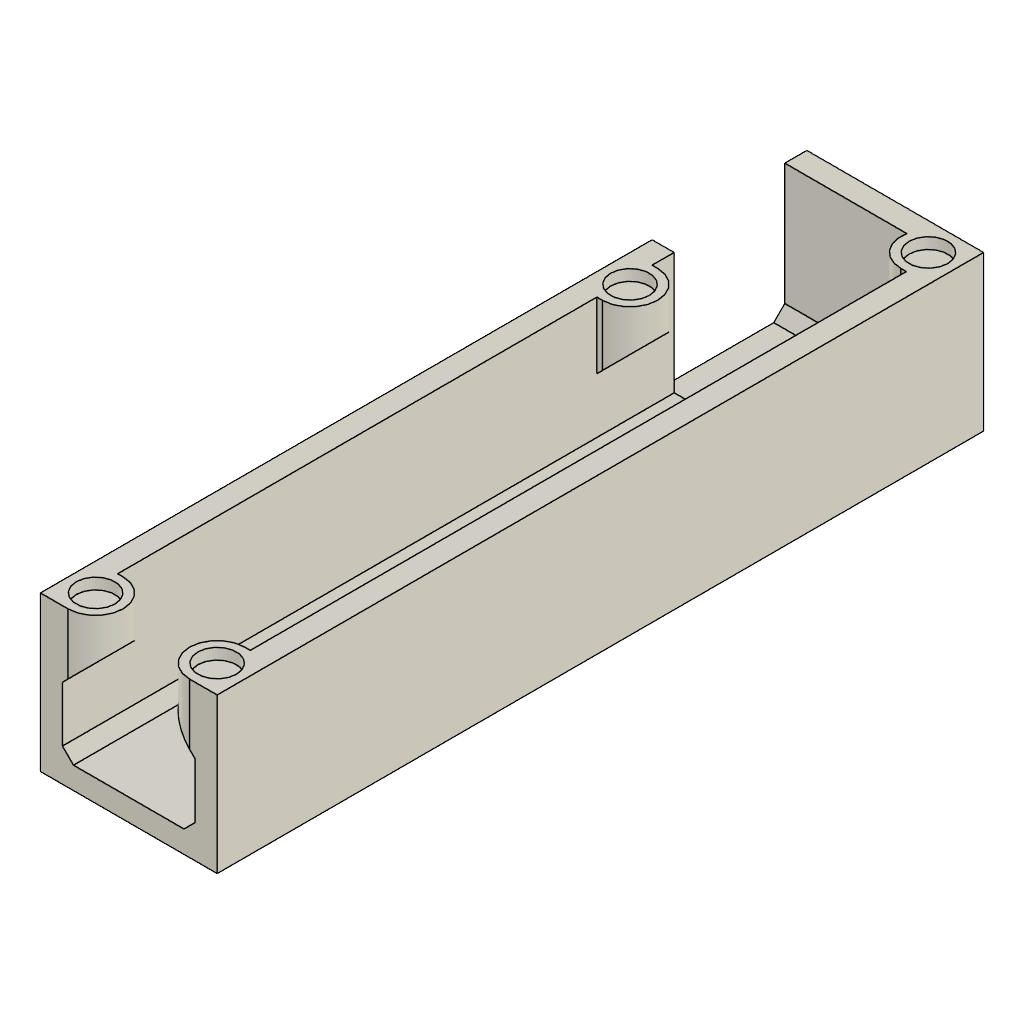
smartie_hopper_mechanism_conduit_1 (Autodesk Fusion 360 archive; units mm, degrees)
design "Smartie Hopper Mechanism Conduit 1 Bottom"
part number: 2026-09-19-14-55-36-645
Autodesk Fusion 360 part; units mm, degrees
note: some values were not read from the file. Set by a fixed rule: which sketch regions a step uses.
sketch "3D-printed conduit outline" plane through (0, 0, 0) normal (0, 1, 0) x (1, 0, 0)
  line L0 (0, 0) -> (16, 0)
  line L1 (16, 0) -> (16, -14)
  line L2 (16, -14) -> (0, -14)
  line L3 (0, -14) -> (0, 0)
  line L4 (2, -14) -> (14, -14)
  line L5 (14, -14) -> (14, -2)
  line L6 (14, -2) -> (2, -2)
  line L7 (2, -2) -> (2, -14)
  dimension "d8" = 14
  dimension "d9" = 16
  dimension "d10" = 2
  dimension "d11" = 2
  dimension "d12" = 2
  constraint horizontal L0
  constraint vertical L1
  constraint horizontal L2
  constraint vertical L3
  constraint coincident L0.start L3.end
  constraint horizontal L4
  constraint vertical L5
  constraint horizontal L6
  constraint vertical L7
  constraint coincident L2 L4.start
  measures "d8" distance of L0.start L2.end
  measures "d9" distance of L0.start L0.end
  measures "d10" distance of L1 L5
  measures "d11" distance of L3 L7
  measures "d12" distance of L0 L6
extrude "Extrude1" add sketch "3D-printed conduit outline" along normal blind 69.355 contours L0 L1 L2 L3 L5 L6 L7
sketch "Magnet holders" plane through (0, 0, 14) normal (0, 0, 1) x (-1, 0, 0)
  line L0 (0, 0) -> (-2, 0)
  line L1 (-2, 0) -> (-2, -69.355)
  line L2 (-2, -69.355) -> (0, -69.355)
  line L3 (0, -69.355) -> (0, 0)
  line L4 (-14, 0) -> (-16, 0)
  line L5 (-16, 0) -> (-16, -69.355)
  line L6 (-16, -69.355) -> (-14, -69.355)
  line L7 (-14, -69.355) -> (-14, 0)
  circle A0 centre (-2.5, -2.5) radius 2.5
  circle A1 centre (-2.5, -2.5) radius 1.75
  line L8 (-14, 0) -> (-2, 0)
  line L9 (0, 0) -> (-2.5, 0)
  line L10 (-2.5, 0) -> (-2.5, -5)
  line L11 (-2.5, -5) -> (0, -5)
  line L12 (0, -5) -> (0, 0)
  circle A2 centre (-13.5, -2.5) radius 2.5
  circle A3 centre (-13.5, -2.5) radius 1.75
  line L13 (-16, 0) -> (-13.5, 0)
  line L14 (-13.5, 0) -> (-13.5, -5)
  line L15 (-13.5, -5) -> (-16, -5)
  line L16 (-16, -5) -> (-16, 0)
  circle A4 centre (-2.5, -50.855) radius 1.75
  circle A5 centre (-2.5, -50.855) radius 2.5
  line L17 (-2.5, -48.355) -> (-2.5, -53.355)
  line L18 (-2.5, -53.355) -> (0, -53.355)
  line L19 (0, -53.355) -> (0, -48.355)
  line L20 (0, -48.355) -> (-2.5, -48.355)
  circle A6 centre (-13.5, -66.855) radius 2.5
  circle A7 centre (-13.5, -66.855) radius 1.75
  line L21 (-13.5, -64.355) -> (-13.5, -69.355)
  line L22 (-13.5, -69.355) -> (-16, -69.355)
  line L23 (-16, -69.355) -> (-16, -64.355)
  line L24 (-16, -64.355) -> (-13.5, -64.355)
  dimension "d15" = 5
  dimension "d16" = 3.5
  dimension "d17" = 5
  dimension "d18" = 3.5
  dimension "d21" = 0
  dimension "d22" = -48.355
  dimension "d42" = 0
  dimension "d43" = -64.355
  constraint concentric A0 A1
  constraint tangent A0 L8
  constraint tangent L3 A0
  constraint horizontal L9
  constraint vertical L10
  constraint horizontal L11
  constraint vertical L12
  constraint coincident L0.start L3.end
  constraint tangent A0 L11
  constraint coincident A0 L9.end
  constraint concentric A2 A3
  constraint tangent L5 A2
  constraint tangent L8 A2
  constraint horizontal L13
  constraint vertical L14
  constraint horizontal L15
  constraint vertical L16
  constraint coincident L4.end L5.start
  constraint tangent A2 L15
  constraint coincident A2 L13.end
  measures "d15" diameter of A0
  measures "d16" diameter of A1
  measures "d17" diameter of A2
  measures "d18" diameter of A3
sketch "End wall" plane through (0, 69.355, 0) normal (0, 1, 0) x (-1, 0, 0)
  line L0 (-2, 2) -> (-14, 2)
  line L1 (-14, 2) -> (-14, 14)
  line L2 (-14, 14) -> (-16, 14)
  line L3 (-16, 14) -> (-16, 0)
  line L4 (-16, 0) -> (0, 0)
  line L5 (0, 0) -> (0, 14)
  line L6 (0, 14) -> (-2, 14)
  line L7 (-2, 14) -> (-2, 2)
  line L8 (-16, 0) -> (0, 0)
  line L9 (0, 0) -> (0, 14)
  line L10 (0, 14) -> (-16, 14)
  line L11 (-16, 14) -> (-16, 0)
  constraint horizontal L8
  constraint vertical L9
  constraint horizontal L10
  constraint vertical L11
  constraint coincident L5.end L6.start
  constraint coincident L3.end L4.start
extrude "Extrude8" add sketch "End wall" against normal blind 2
extrude "Extrude2" add sketch "Magnet holders" against normal blind 3 contours L1 A0 L8 L9 | L1 A0 A1 L10 | A0 A1 L10 | L1 A0 A1 L10 | L1 A0 L11 | L1 A1 L10 | A1 L10 | L1 A5 L20 | L1 A4 A5 L17 | L1 A4 A5 L17 | L1 A5 L18 | A4 A5 L17 | L1 A4 L17 | A4 L17 | L7 L8 A2 L13 | L7 A2 A3 L14 | A2 A3 L14 | L7 A3 L14 | A3 L14 | L7 A2 L15 | L7 A2 A3 L14 | L7 A6 L24 | L7 A6 A7 L21 | L7 A6 L22 | L7 A6 A7 L21 | A6 A7 L21 | L7 A7 L21 | A7 L21
extrude "Extrude4" cut sketch "Magnet holders" against normal blind 1 contours L1 A1 | L1 A1 L10 | A1 L10 | L1 A4 | L1 A4 L17 | A4 L17 | L7 A3 L14 | L7 A3 | A3 L14 | L7 A7 L21 | L7 A7 | A7 L21
chamfer "Chamfer2" distance 2.9999 angle 45 5 edges at (2, 2.5, 11) (2, 50.855, 11) (2, 2.5, 11) (14, 2.5, 11) (14, 65.855, 11)
sketch "Smartie hopper mechanism conduit 2 outlet" plane through (0, 0, 0) normal (-1, 0, 0) x (0, -1, 0)
  line L0 (-69.355, 0) -> (0, 0)
  line L1 (0, 0) -> (0, 14)
  line L2 (0, 14) -> (-69.355, 14)
  line L3 (-69.355, 14) -> (-69.355, 0)
  line L4 (-67.355, 14) -> (-55.355, 14)
  line L5 (-55.355, 14) -> (-55.355, 2)
  line L6 (-55.355, 2) -> (-67.355, 2)
  line L7 (-67.355, 2) -> (-67.355, 14)
  dimension "d60" = 2
  dimension "d61" = 12
  dimension "d62" = 2
  constraint horizontal L4
  constraint vertical L5
  constraint horizontal L6
  constraint vertical L7
  constraint coincident L2 L4.start
  measures "d60" distance of L3 L7
  measures "d61" distance of L5 L7
  measures "d62" distance of L0 L6
extrude "Extrude11" cut sketch "Smartie hopper mechanism conduit 2 outlet" against normal blind 2 contours L2 L4 L5 L6 L7
chamfer "Chamfer5" distance 1 angle 45 4 edges at (2, 27.6775, 2) (1, 55.355, 2) (7, 67.355, 2) (14, 33.6775, 2)
equation "conduit_length = 69.355 mm"
equation "conduit_width = 16 mm"
equation "conduit_height = 16 mm"
equation "conduit_wall_thickness = 2 mm"
equation "magnet_diameter = 3 mm"
equation "magnet_height = 1 mm"
equation "number_of_magnets_on_a_side = 2"
equation "d8 = conduit_height - conduit_wall_thickness"
equation "d9 = conduit_width"
equation "d10 = conduit_wall_thickness"
equation "d11 = conduit_wall_thickness"
equation "d12 = conduit_wall_thickness"
equation "d13 = conduit_length"
equation "d15 = magnet_diameter + 2 mm"
equation "d16 = magnet_diameter + 0.5 mm"
equation "d17 = magnet_diameter + 2 mm"
equation "d18 = magnet_diameter + 0.5 mm"
equation "d20 = number_of_magnets_on_a_side"
equation "d22 = -conduit_length + ( magnet_diameter + 2 mm ) + ( conduit_width )"
equation "d23 = -( magnet_height + 2 mm )"
equation "d29 = -magnet_height"
equation "d41 = number_of_magnets_on_a_side"
equation "d43 = -conduit_length + ( magnet_diameter + 2 mm )"
equation "d46 = -conduit_wall_thickness"
equation "d60 = conduit_wall_thickness"
equation "d62 = conduit_wall_thickness"
equation "d63 = -conduit_wall_thickness"
equation "d48 = conduit_wall_thickness"
equation "d49 = conduit_wall_thickness"
equation "d50 = conduit_width - 2 * conduit_wall_thickness"
equation "d54 = conduit_wall_thickness"
named bodies: "Smartie hopper mechanism conduit 1 bottom"

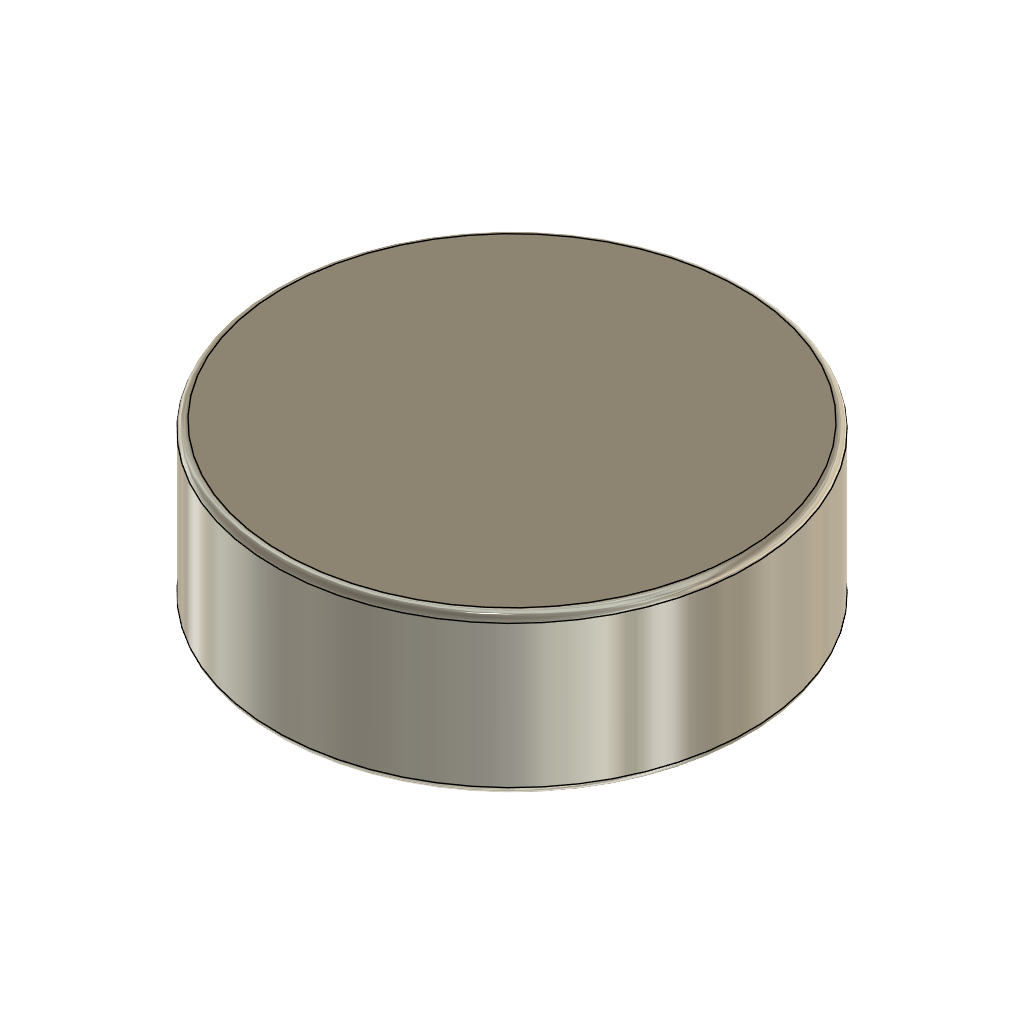
design "3 mm x 1 mm Neodymium Disc Magnet"
Autodesk Fusion 360 part; units mm, degrees
sketch "3 mm x 1 mm neodymium disc magnet" plane through (0, 0, 0) normal (0, 0, 1) x (1, 0, 0)
  circle A0 centre (0, 0) radius 1.5
  dimension "d1" = 3
  constraint coincident A0.centre origin
  measures "d1" diameter of A0
extrude "Extrude1" add sketch "3 mm x 1 mm neodymium disc magnet" along normal blind 1
fillet "Fillet1" radius 0.05 2 edges at (-1.3985, -0.5424, 1) (-1.3985, -0.5424, 0)
named bodies: "3 mm x 1 mm Neodymium Disc Magnet"

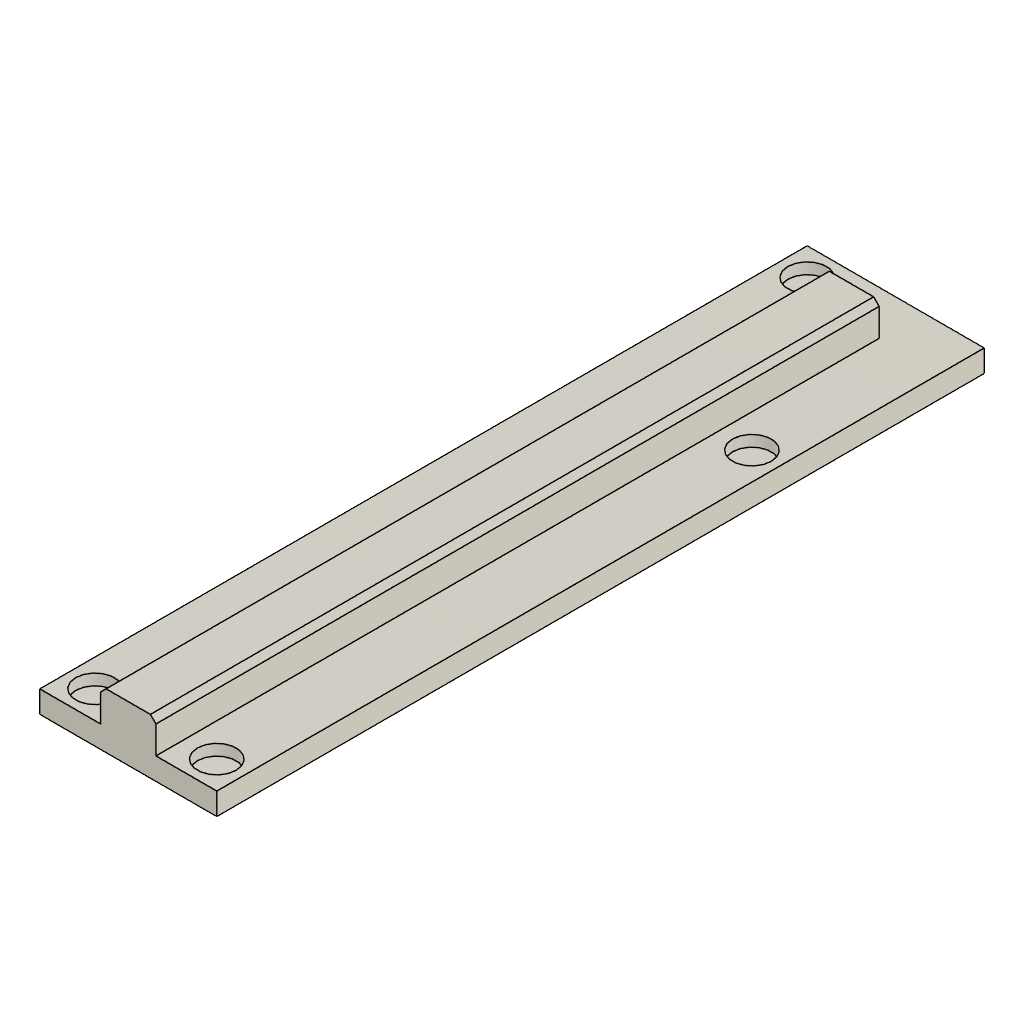
design "Smartie Hopper Mechanism Conduit 1 Top"
part number: 2026-09-19-15-15-46-900
Autodesk Fusion 360 part; units mm, degrees
sketch "3D-printed conduit top outline" plane through (0, 0, 0) normal (0, 1, 0) x (1, 0, 0)
  line L0 (0, 0) -> (16, 0)
  line L1 (16, 0) -> (16, -2)
  line L2 (16, -2) -> (0, -2)
  line L3 (0, -2) -> (0, 0)
  dimension "d7" = 16
  dimension "d8" = 2
  constraint horizontal L0
  constraint vertical L1
  constraint horizontal L2
  constraint vertical L3
  constraint coincident L0.start L3.end
  measures "d7" distance of L0.start L0.end
  measures "d8" distance of L0.start L2.end
extrude "Extrude1" add sketch "3D-printed conduit top outline" along normal blind 69.355
sketch "Magnet holes" plane through (0, 0, 2) normal (0, 0, 1) x (-1, 0, 0)
  line L0 (0, 0) -> (-16, 0)
  line L1 (-16, 0) -> (-16, -69.355)
  line L2 (-16, -69.355) -> (0, -69.355)
  line L3 (0, -69.355) -> (0, 0)
  circle A0 centre (-2.5, -2.5) radius 2.5
  circle A1 centre (-13.5, -2.5) radius 2.5
  circle A2 centre (-2.5, -2.5) radius 1.75
  circle A3 centre (-13.5, -2.5) radius 1.75
  circle A4 centre (-2.5, -66.855) radius 1.75
  circle A5 centre (-2.5, -66.855) radius 2.5
  circle A6 centre (-13.5, -50.855) radius 2.5
  circle A7 centre (-13.5, -50.855) radius 1.75
  dimension "d11" = 5
  dimension "d12" = 5
  dimension "d13" = 3.5
  dimension "d14" = 3.5
  dimension "d17" = 0
  dimension "d18" = -64.355
  dimension "d32" = 0
  dimension "d33" = -48.355
  constraint concentric A0 A2
  constraint concentric A1 A3
  constraint tangent L3 A0
  constraint tangent L0 A0
  constraint tangent L1 A1
  constraint tangent L0 A1
  measures "d11" diameter of A0
  measures "d12" diameter of A1
  measures "d13" diameter of A2
  measures "d14" diameter of A3
extrude "Extrude4" cut sketch "Magnet holes" against normal blind 1 contours A2 | A3 | A4 | A7
sketch "Support rib" plane through (0, 0, 2) normal (0, 0, 1) x (-1, 0, 0)
  circle A0 centre (-13.5, -2.5) radius 1.75
  circle A1 centre (-2.5, -66.855) radius 1.75
  circle A2 centre (-2.5, -2.5) radius 1.75
  circle A3 centre (-13.5, -50.855) radius 1.75
  line L0 (0, 0) -> (-16, 0)
  line L1 (-16, 0) -> (-16, -69.355)
  line L2 (-16, -69.355) -> (0, -69.355)
  line L3 (0, -69.355) -> (0, 0)
  line L4 (-5.5, 0) -> (-10.5, 0)
  line L5 (-10.5, 0) -> (-10.5, -65.355)
  line L6 (-10.5, -65.355) -> (-5.5, -65.355)
  line L7 (-5.5, -65.355) -> (-5.5, 0)
  dimension "d36" = 5
  dimension "d37" = 5.5
  dimension "d38" = 5.5
  dimension "d39" = 4
  constraint horizontal L4
  constraint vertical L5
  constraint horizontal L6
  constraint vertical L7
  constraint coincident L0 L4.start
  measures "d36" distance of L5 L7
  measures "d37" distance of L3 L7
  measures "d38" distance of L1 L5
  measures "d39" distance of L2 L6
extrude "Extrude3" add sketch "Support rib" along normal blind 3 contours L0 L4 L5 L6 L7
chamfer "Chamfer2" distance 0.5 angle 45 2 edges at (10.5, 32.6775, 5) (5.5, 32.6775, 5)
equation "conduit_length = 69.355 mm"
equation "conduit_width = 16 mm"
equation "conduit_wall_thickness = 2 mm"
equation "magnet_diameter = 3 mm"
equation "magnet_height = 1 mm"
equation "number_of_magnets_on_a_side = 2"
equation "d7 = conduit_width"
equation "d8 = conduit_wall_thickness"
equation "d9 = conduit_length"
equation "d11 = magnet_diameter + 2 mm"
equation "d12 = magnet_diameter + 2 mm"
equation "d13 = magnet_diameter + 0.5 mm"
equation "d14 = magnet_diameter + 0.5 mm"
equation "d16 = number_of_magnets_on_a_side"
equation "d18 = -conduit_length + ( magnet_diameter + 2 mm )"
equation "rib_width = 5 mm"
equation "rib_height = 3 mm"
equation "d26 = rib_height"
equation "rib_chamfer = 0.5 mm"
equation "d31 = number_of_magnets_on_a_side"
equation "d33 = -conduit_length + ( magnet_diameter + 2 mm ) + ( conduit_width )"
equation "d34 = -magnet_height"
equation "d36 = rib_width"
equation "d37 = ( conduit_width - rib_width ) / 2"
equation "d39 = 2 * conduit_wall_thickness"
equation "d40 = rib_chamfer"
equation "d29 = rib_fillet"
named bodies: "Smartie hopper mechanism conduit 1 top"
